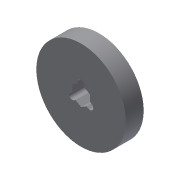
# Autodesk Inventor part: augmented gear v3
Saved by Autodesk Inventor 2014 (Build 180170000, 170)
## iProperties
Created: 2014-02-23
Part Number: augmented gear v3
Material: Generic
Document SubType Name: Modeling
Designer: Owner
Density: 1 g/cm^3
Appearance: Default
Author: Owner
Autodesk Inventor part; units mm, degrees
ref_plane "YZ Plane" through (0, 0, 0) normal (1, 0, 0) x (0, 1, 0)
ref_plane "XZ Plane" through (0, 0, 0) normal (0, 1, 0) x (-1, 0, 0)
ref_plane "XY Plane" through (0, 0, 0) normal (0, 0, 1) x (1, 0, 0)
sketch "Sketch1" plane through (0, 0, 0) normal (0, 0, 1) x (1, 0, 0)
  line L0 (0, 0) -> (0, 7.239) construction
  line L1 (0, 0) -> (6.2692, 3.6195) construction
  line L2 (0, 0) -> (6.2692, -3.6195) construction
  line L3 (0, 0) -> (0, -7.239) construction
  line L4 (0, 0) -> (-6.2692, -3.6195) construction
  line L5 (0, 0) -> (-6.2692, 3.6195) construction
  line L6 (0, 7.239) -> (6.2692, 3.6195)
  line L7 (6.2692, 3.6195) -> (6.2692, -3.6195)
  line L8 (6.2692, -3.6195) -> (0, -7.239)
  line L9 (0, -7.239) -> (-6.2692, -3.6195)
  line L10 (-6.2692, -3.6195) -> (-6.2692, 3.6195)
  line L11 (-6.2692, 3.6195) -> (0, 7.239)
  circle A0 centre (0, 7.239) radius 2.3813
  circle A1 centre (6.2692, -3.6195) radius 2.3813
  circle A2 centre (-6.2692, -3.6195) radius 2.3813
  circle A3 centre (0, 0) radius 31.75
  line L12 (-2.3813, 7.239) -> (-2.3813, 5.8642)
  line L13 (2.3813, 7.239) -> (2.3812, 5.8642)
  line L14 (-2.3813, 7.239) -> (2.3813, 7.239)
  line L15 (-2.3813, 5.8642) -> (2.3812, 5.8642)
  line L16 (7.4598, -1.5573) -> (6.2692, -0.8699)
  line L17 (5.0785, -5.6817) -> (3.8879, -4.9943)
  line L18 (6.2692, -0.8699) -> (3.8879, -4.9943)
  line L19 (7.4598, -1.5573) -> (5.0785, -5.6817)
  line L20 (-7.4598, -1.5573) -> (-6.2692, -0.8699)
  line L21 (-5.0785, -5.6817) -> (-3.8879, -4.9943)
  line L22 (-7.4598, -1.5573) -> (-5.0785, -5.6817)
  line L23 (-3.8879, -4.9943) -> (-6.2692, -0.8699)
  dimension "d0" = 7.239
  dimension "d1" = 60
  dimension "d2" = 60
  dimension "d3" = 4.7625
  dimension "d4" = 4.7625
  dimension "d5" = 4.7625
  dimension "d6" = 63.5
  constraints: 48 end point, 8 parallel, 7 point on circle, 6 point on line, 6 tangent, 5 equal length, 4 centre point, 4 coincident, 3 collinear, 1 perpendicular, 1 vertical
  measures "d0" distance of L0.start L0.end
  measures "d1" angle of L0 L1
  measures "d2" angle of L2 L1
  measures "d3" diameter of A0
  measures "d4" diameter of A1
  measures "d5" diameter of A2
  measures "d6" diameter of A3
extrude "Extrusion1" add sketch "Sketch1" along normal blind 12.7 contours L6 A0 L13 | L16 A1 L7 | A0 L11 L12 | A1 L17 L8 | L10 A2 L20 | L21 A2 L9 | A3
extrude "Extrusion2" cut sketch "Sketch1" along normal blind 12.7 contours L6 A0 L13 | L6 L7 L18 A1 L8 L9 L23 A2 L10 L11 L15 A0 | L6 L14 A0 | A0 L15 | L7 A1 L18 | L11 A0 L14 | A0 L11 L12 | L7 L8 A1 L18 | L18 A1 | A1 L8 L18 | L23 A2 L10 | A2 L23 L9 L10 | A2 L23 | L9 A2 L23
extrude "Extrusion3" cut sketch "Sketch1" along normal blind 12.7 contours L16 A1 L7 | A1 L19 L7 | A1 L19 | L19 A1 L8 | A1 L17 L8
extrude "Extrusion4" cut sketch "Sketch1" along normal through all contours L10 A2 L20 | L10 L22 A2 | L21 A2 L9 | L9 A2 L22
equation "\"d4\" = d3"
equation "\"d5\" = d3"
body "Solid1"
